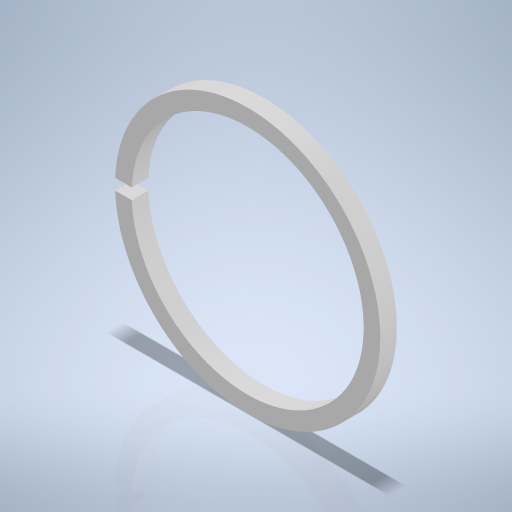
# Autodesk Inventor part: kolbenring
Saved by Autodesk Inventor 2024 (Build 280153000, 153)
## iProperties
Created: 2024-04-30
Part Number: kolbenring
Material: Generisch
Document SubType Name: Modeling
Designer: ffogue
Density: 1 g/cm^3
Appearance: Vorgabe
Author: ffogue
Autodesk Inventor part; units mm, degrees
ref_plane "YZ Plane" through (0, 0, 0) normal (1, 0, 0) x (0, 1, 0)
ref_plane "XZ Plane" through (0, 0, 0) normal (0, 1, 0) x (-1, 0, 0)
ref_plane "XY Plane" through (0, 0, 0) normal (0, 0, 1) x (1, 0, 0)
sketch "Skizze1" plane through (0, 0, 0) normal (0, 1, 0) x (-1, 0, 0)
  circle A0 centre (0, 0) radius 10.5
  circle A1 centre (0, 0) radius 12
  dimension "d0" = 21
  dimension "d1" = 24
  constraints: 2 centre point, 2 coincident
  measures "d0" diameter of A0
  measures "d1" diameter of A1
extrude "Extrusion1" add sketch "Skizze1" along normal blind 1.5
sketch "Skizze2" plane through (0, 1.5, 0) normal (0, 1, 0) x (1, 0, 0)
  circle A0 centre (0, 0) radius 12 projected
  circle A1 centre (0, 0) radius 10.5 projected
  line L0 (-10.4881, -0.5) -> (-11.9896, -0.5)
  line L1 (-11.9896, 0.5) -> (-10.4881, 0.5)
  line L2 (0, 0) -> (-4.204, 0) construction
  dimension "d4" = 1
  constraints: 6 end point, 4 point on circle, 2 horizontal, 1 parallel, 1 other
  measures "d4" distance between parallel lines of L1 L0
extrude "Extrusion2" cut sketch "Skizze2" against normal up to surface (1.5 mm away) contours L1 A1 L0 A0 picked at (-10.9921, -0.3889)
